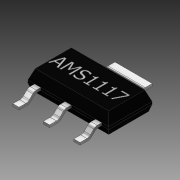
# Autodesk Inventor part: AMS1117
Saved by Autodesk Inventor 2015 SP1 (Build 190203100, 203)
## iProperties
Created: 2016-08-04
Part Number: AMS1117
Material: Generisch
Document SubType Name: Modeling
Designer: Gabriel
Density: 1 g/cm^3
Appearance: Vorgabe
Author: Gabriel
Autodesk Inventor part; units mm, degrees
ref_plane "YZ Plane" through (0, 0, 0) normal (1, 0, 0) x (0, 1, 0)
ref_plane "XZ Plane" through (0, 0, 0) normal (0, 1, 0) x (-1, 0, 0)
ref_plane "XY Plane" through (0, 0, 0) normal (0, 0, 1) x (1, 0, 0)
sketch "Skizze1" plane through (0, 0, 0) normal (0, 0, 1) x (1, 0, 0)
  line L0 (-3.25, -1.75) -> (3.25, -1.75)
  line L1 (3.25, -1.75) -> (3.25, 1.75)
  line L2 (3.25, 1.75) -> (-3.25, 1.75)
  line L3 (-3.25, 1.75) -> (-3.25, -1.75)
  line L4 (-3.25, -1.75) -> (3.25, 1.75) construction
  line L5 (3.25, -1.75) -> (-3.25, 1.75) construction
  point P0 (0, 0)
  dimension "d0" = 6.5
  dimension "d1" = 3.5
  constraints: 12 end point, 2 midpoint, 2 parallel, 1 horizontal, 1 perpendicular
  measures "d0" distance of L2.end L1.end
  measures "d1" distance of L1.end L0.end
extrude "Extrusion1" add sketch "Skizze1" along normal blind 1.5
sketch "Skizze2" plane through (3.25, -1.75, 0) normal (1, 0, 0) x (0, 0, -1)
  line L0 (0, 3.5) -> (-1.5, 3.5) projected
  line L1 (-0.7, 3.5) -> (-0.7, 4.0328)
  line L2 (-0.7, 4.0328) -> (-0.2, 4.5328)
  line L3 (-0.2, 4.5328) -> (-0.2, 5.25)
  line L4 (-0.2, 5.25) -> (0, 5.25)
  line L5 (0, 5.25) -> (0, 4.45)
  line L6 (0, 4.45) -> (-0.5, 3.95)
  line L7 (-0.5, 3.95) -> (-0.5, 3.5)
  line L8 (0, 0) -> (0, 3.5) projected
  point P0 (0, 1.75)
  dimension "d4" = 0.8
  dimension "d5" = 0.7
  dimension "d6" = 0.2
  dimension "d7" = 0.2
  dimension "d8" = 0.2
  dimension "d9" = 1.75
  dimension "d10" = 45
  constraints: 14 end point, 3 parallel, 3 perpendicular, 2 point on line, 1 collinear
  measures "d4" distance of L4.end L5.end
  measures "d5" distance between parallel lines of L8 L1
  measures "d6" distance of L3.end L4.end
  measures "d7" distance between parallel lines of L2 L6
  measures "d8" distance between parallel lines of L1 L7
  measures "d9" distance between parallel lines of L0 L4
  measures "d10" angle of L0 L6
extrude "Extrusion2" add sketch "Skizze2" against normal blind 6.5
mirror "Spiegeln1" about plane through (0, 0, 0) normal (0, 1, 0) of "Extrusion2"
sketch "Skizze3" plane through (0, 0, 1.5) normal (0, 0, 1) x (1, 0, 0)
  line L0 (-3.25, 3.5) -> (-1.5, 3.5)
  line L1 (-1.5, 3.5) -> (-1.5, 1.75)
  line L2 (-1.5, 1.75) -> (-3.25, 1.75)
  line L3 (-3.25, 1.75) -> (-3.25, 3.5)
  line L4 (1.5, 3.5) -> (3.25, 3.5)
  line L5 (3.25, 3.5) -> (3.25, 1.75)
  line L6 (3.25, 1.75) -> (1.5, 1.75)
  line L7 (1.5, 1.75) -> (1.5, 3.5)
  line L8 (-3.25, -3.5) -> (-2.7, -3.5)
  line L9 (-2.7, -3.5) -> (-2.7, -1.75)
  line L10 (-2.7, -1.75) -> (-3.25, -1.75)
  line L11 (-3.25, -1.75) -> (-3.25, -3.5)
  line L12 (-0.25, -3.5) -> (-2.2, -3.5)
  line L13 (-2.2, -3.5) -> (-2.2, -1.75)
  line L14 (-2.2, -1.75) -> (-0.25, -1.75)
  line L15 (-0.25, -1.75) -> (-0.25, -3.5)
  line L16 (0.25, -1.75) -> (2.2, -1.75)
  line L17 (2.2, -1.75) -> (2.2, -3.5)
  line L18 (2.2, -3.5) -> (0.25, -3.5)
  line L19 (0.25, -3.5) -> (0.25, -1.75)
  line L20 (2.7, -3.5) -> (3.25, -3.5)
  line L21 (3.25, -3.5) -> (3.25, -1.75)
  line L22 (3.25, -1.75) -> (2.7, -1.75)
  line L23 (2.7, -1.75) -> (2.7, -3.5)
  line L24 (-3.25, -1.75) -> (3.25, -1.75) projected
  line L25 (3.25, 3.5) -> (-3.25, 3.5) projected
  line L26 (3.25, 1.75) -> (-3.25, 1.75) projected
  line L27 (3.25, 3.5) -> (3.25, 2.7828) projected
  line L28 (-3.25, 2.7828) -> (-3.25, 3.5) projected
  line L29 (0, 5.1518) -> (0, -6.0635) construction
  line L30 (3.25, -2.2828) -> (3.25, -1.75) construction
  line L31 (3.25, -3.5) -> (-3.25, -3.5) construction
  point P0 (0, 0)
  dimension "d13" = 3
  dimension "d14" = 0.5
  dimension "d15" = 5.4
  dimension "d16" = 0.5
  constraints: 50 end point, 18 perpendicular, 15 collinear, 6 horizontal, 1 point on line, 1 vertical, 5 other
  measures "d13" distance between parallel lines of L1 L7
  measures "d14" distance between parallel lines of L15 L19
  measures "d15" distance between parallel lines of L23 L9
  measures "d16" distance between parallel lines of L9 L13
extrude "Extrusion3" cut sketch "Skizze3" against normal blind 6.5 contours L0 L1 L2 L3 | L4 L5 L6 L7 | L11 L10 L9 L8 | L22 L21 L20 L23 | L16 L17 L18 L19 | L14 L15 L12 L13
chamfer "Fase1" distance 0.3 distance2 0.8 1 edges at (0, 1.75, 1.5) measured on face at (1.0833, -0.5833, 1.5)
chamfer "Fase2" distance 0.3 distance2 0.8 1 edges at (0, -1.75, 1.5) measured on face at (-1.0833, 0.3837, 1.5)
chamfer "Fase3" distance 0.5 distance2 0.15 1 edges at (0, 1.75, 0) measured on face at (0.5, 1.75, 0.1667)
chamfer "Fase4" distance 0.5 distance2 0.15 1 edges at (0, -1.75, 0) measured on face at (-0.0833, -1.75, 0.1667)
fillet "Rundung1" radius 0.4 16 edges at (2.45, -2.2828, 0.7) (2.45, -2.2, 0.5) (2.45, -2.7, 0) (2.45, -2.7828, 0.2) (0, -2.2, 0.5) (0, -2.7, 0) (0, -2.2828, 0.7) (0, -2.7828, 0.2) (-2.45, -2.2828, 0.7) (-2.45, -2.2, 0.5) (-2.45, -2.7, 0) (-2.45, -2.7828, 0.2) (0, 2.7, 0) (0, 2.7828, 0.2) (0, 2.2, 0.5) (0, 2.2828, 0.7)
sketch "Skizze4" plane through (0, 0, 1.5) normal (0, 0, 1) x (1, 0, 0)
  line L0 (-2.8892, 0.5274) -> (2.8892, 0.5274) construction
  line L1 (2.8892, 0.5274) -> (2.8892, -0.5274) construction
  line L2 (2.8892, -0.5274) -> (-2.8892, -0.5274) construction
  line L3 (-2.8892, -0.5274) -> (-2.8892, 0.5274) construction
  line L4 (-2.8957, -0.4904) -> (-2.5585, 0.5096)
  line L5 (-2.5585, 0.5096) -> (-2.3948, 0.5096)
  line L6 (-2.3948, 0.5096) -> (-2.0577, -0.4904)
  line L7 (-2.0577, -0.4904) -> (-2.1979, -0.4904)
  line L8 (-2.1979, -0.4904) -> (-2.2887, -0.2108)
  line L9 (-2.2887, -0.2108) -> (-2.6704, -0.2108)
  line L10 (-2.6704, -0.2108) -> (-2.7611, -0.4904)
  line L11 (-2.7611, -0.4904) -> (-2.8957, -0.4904)
  line L12 (-2.3252, -0.0974) -> (-2.4799, 0.3735)
  line L13 (-2.4799, 0.3735) -> (-2.6339, -0.0974)
  line L14 (-2.6339, -0.0974) -> (-2.3252, -0.0974)
  line L15 (-1.1055, -0.4904) -> (-1.2384, -0.4904)
  line L16 (-1.2384, -0.4904) -> (-1.2384, 0.371)
  line L17 (-1.2384, 0.371) -> (-1.4994, -0.2149)
  line L18 (-1.4994, -0.2149) -> (-1.5804, -0.2149)
  line L19 (-1.5804, -0.2149) -> (-1.8389, 0.371)
  line L20 (-1.8389, 0.371) -> (-1.8389, -0.4904)
  line L21 (-1.8389, -0.4904) -> (-1.9629, -0.4904)
  line L22 (-1.9629, -0.4904) -> (-1.9629, 0.5096)
  line L23 (-1.9629, 0.5096) -> (-1.7814, 0.5096)
  line L24 (-1.7814, 0.5096) -> (-1.5318, -0.0471)
  line L25 (-1.5318, -0.0471) -> (-1.2903, 0.5096)
  line L26 (-1.2903, 0.5096) -> (-1.1055, 0.5096)
  line L27 (-1.1055, 0.5096) -> (-1.1055, -0.4904)
  spline S0 degree 2 poles (-0.6242, -0.5082) (-0.7328, -0.5082) (-0.8851, -0.4628) (-0.9524, -0.4304) knots 0 0 0 1 2 2 2
  line L28 (-0.9524, -0.4304) -> (-0.9524, -0.2635)
  line L29 (-0.9524, -0.2635) -> (-0.9427, -0.2635)
  spline S1 degree 2 poles (-0.9427, -0.2635) (-0.877, -0.3251) (-0.7109, -0.3932) (-0.6339, -0.3932) knots 0 0 0 1 2 2 2
  spline S2 degree 2 poles (-0.6339, -0.3932) (-0.5237, -0.3932) (-0.4111, -0.3016) (-0.4111, -0.2262) knots 0 0 0 1 2 2 2
  spline S3 degree 2 poles (-0.4111, -0.2262) (-0.4111, -0.1663) (-0.4702, -0.0917) (-0.5342, -0.0731) knots 0 0 0 1 2 2 2
  spline S4 degree 2 poles (-0.5342, -0.0731) (-0.5804, -0.0601) (-0.6574, -0.0423) (-0.7149, -0.0277) knots 0 0 0 1 2 2 2
  spline S5 degree 2 poles (-0.7149, -0.0277) (-0.7668, -0.0139) (-0.8487, 0.0274) (-0.8803, 0.0607) knots 0 0 0 1 2 2 2
  spline S6 degree 2 poles (-0.8803, 0.0607) (-0.9111, 0.0939) (-0.9451, 0.183) (-0.9451, 0.2414) knots 0 0 0 1 2 2 2
  spline S7 degree 2 poles (-0.9451, 0.2414) (-0.9451, 0.3629) (-0.7555, 0.5274) (-0.6088, 0.5274) knots 0 0 0 1 2 2 2
  spline S8 degree 2 poles (-0.6088, 0.5274) (-0.5245, 0.5274) (-0.3754, 0.4942) (-0.3114, 0.4626) knots 0 0 0 1 2 2 2
  line L30 (-0.3114, 0.4626) -> (-0.3114, 0.3038)
  line L31 (-0.3114, 0.3038) -> (-0.3211, 0.3038)
  spline S9 degree 2 poles (-0.3211, 0.3038) (-0.3689, 0.3475) (-0.518, 0.4124) (-0.5999, 0.4124) knots 0 0 0 1 2 2 2
  spline S10 degree 2 poles (-0.5999, 0.4124) (-0.6923, 0.4124) (-0.8065, 0.3256) (-0.8065, 0.2551) knots 0 0 0 1 2 2 2
  spline S11 degree 2 poles (-0.8065, 0.2551) (-0.8065, 0.1919) (-0.7393, 0.1166) (-0.676, 0.0995) knots 0 0 0 1 2 2 2
  spline S12 degree 2 poles (-0.676, 0.0995) (-0.6339, 0.0882) (-0.5115, 0.059) (-0.471, 0.0469) knots 0 0 0 1 2 2 2
  spline S13 degree 2 poles (-0.471, 0.0469) (-0.3681, 0.0153) (-0.2725, -0.112) (-0.2725, -0.2052) knots 0 0 0 1 2 2 2
  spline S14 degree 2 poles (-0.2725, -0.2052) (-0.2725, -0.2643) (-0.3203, -0.3778) (-0.3632, -0.4175) knots 0 0 0 1 2 2 2
  spline S15 degree 2 poles (-0.3632, -0.4175) (-0.4111, -0.4612) (-0.5326, -0.5082) (-0.6242, -0.5082) knots 0 0 0 1 2 2 2
  line L32 (0.4009, -0.4904) -> (-0.0869, -0.4904)
  line L33 (-0.0869, -0.4904) -> (-0.0869, -0.3883)
  line L34 (-0.0869, -0.3883) -> (0.0946, -0.3883)
  line L35 (0.0946, -0.3883) -> (0.0946, 0.2819)
  line L36 (0.0946, 0.2819) -> (-0.0869, 0.2819)
  line L37 (-0.0869, 0.2819) -> (-0.0869, 0.3735)
  spline S16 degree 2 poles (-0.0869, 0.3735) (0.016, 0.3735) (0.1133, 0.4318) (0.1197, 0.5128) knots 0 0 0 1 2 2 2
  line L38 (0.1197, 0.5128) -> (0.2235, 0.5128)
  line L39 (0.2235, 0.5128) -> (0.2235, -0.3883)
  line L40 (0.2235, -0.3883) -> (0.4009, -0.3883)
  line L41 (0.4009, -0.3883) -> (0.4009, -0.4904)
  line L42 (1.1513, -0.4904) -> (0.6635, -0.4904)
  line L43 (0.6635, -0.4904) -> (0.6635, -0.3883)
  line L44 (0.6635, -0.3883) -> (0.845, -0.3883)
  line L45 (0.845, -0.3883) -> (0.845, 0.2819)
  line L46 (0.845, 0.2819) -> (0.6635, 0.2819)
  line L47 (0.6635, 0.2819) -> (0.6635, 0.3735)
  spline S17 degree 2 poles (0.6635, 0.3735) (0.7664, 0.3735) (0.8637, 0.4318) (0.8701, 0.5128) knots 0 0 0 1 2 2 2
  line L48 (0.8701, 0.5128) -> (0.9739, 0.5128)
  line L49 (0.9739, 0.5128) -> (0.9739, -0.3883)
  line L50 (0.9739, -0.3883) -> (1.1513, -0.3883)
  line L51 (1.1513, -0.3883) -> (1.1513, -0.4904)
  line L52 (1.9017, -0.4904) -> (1.4139, -0.4904)
  line L53 (1.4139, -0.4904) -> (1.4139, -0.3883)
  line L54 (1.4139, -0.3883) -> (1.5954, -0.3883)
  line L55 (1.5954, -0.3883) -> (1.5954, 0.2819)
  line L56 (1.5954, 0.2819) -> (1.4139, 0.2819)
  line L57 (1.4139, 0.2819) -> (1.4139, 0.3735)
  spline S18 degree 2 poles (1.4139, 0.3735) (1.5168, 0.3735) (1.6141, 0.4318) (1.6205, 0.5128) knots 0 0 0 1 2 2 2
  line L58 (1.6205, 0.5128) -> (1.7243, 0.5128)
  line L59 (1.7243, 0.5128) -> (1.7243, -0.3883)
  line L60 (1.7243, -0.3883) -> (1.9017, -0.3883)
  line L61 (1.9017, -0.3883) -> (1.9017, -0.4904)
  line L62 (2.7137, 0.3597) -> (2.281, -0.4904)
  line L63 (2.281, -0.4904) -> (2.1384, -0.4904)
  line L64 (2.1384, -0.4904) -> (2.5954, 0.3921)
  line L65 (2.5954, 0.3921) -> (2.0792, 0.3921)
  line L66 (2.0792, 0.3921) -> (2.0792, 0.5096)
  line L67 (2.0792, 0.5096) -> (2.7137, 0.5096)
  line L68 (2.7137, 0.5096) -> (2.7137, 0.3597)
  point P0 (0, 0)
  point P1 (-2.8892, 0)
  point P2 (0, 0.5274)
  constraints: 2 midpoint, 1 horizontal alignment, 1 vertical alignment, 2 other
extrude "Extrusion4" cut sketch "Skizze4" against normal blind 0.01
chamfer "Fase5" distance 0.5 distance2 0.15 1 edges at (-3.25, 0, 0) measured on face at (-3.25, 0.4835, 0.5)
chamfer "Fase6" distance 0.5 distance2 0.15 1 edges at (3.25, 0, 0) measured on face at (3.25, -0.4835, 0.5)
chamfer "Fase7" distance 0.3 distance2 0.8 1 edges at (3.25, 0, 1.5) measured on face at (-0.029, -1.1305, 1.5)
chamfer "Fase8" distance 0.3 distance2 0.8 1 edges at (-3.25, 0, 1.5) measured on face at (-0.129, -1.1305, 1.5)
equation "\"d8\" = d7"
